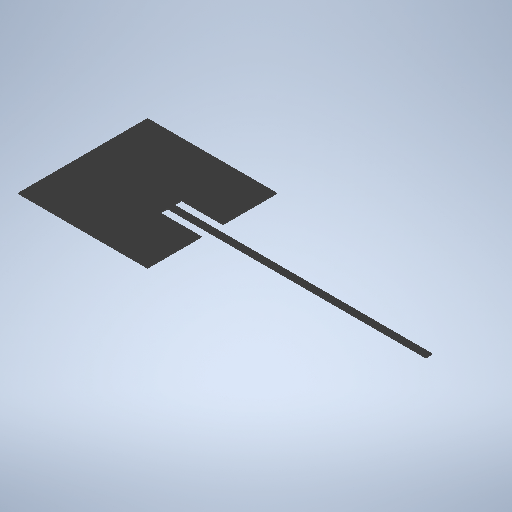
# Autodesk Inventor part: Part17
Saved by Autodesk Inventor 2025.2 (Build 292293000, 293)
## iProperties
Created: 2026-03-30
Part Number: Part17
Material: Generic
Document SubType Name: Modeling
Designer: composite
Density: 1 g/cm^3
Appearance: Default
Author: composite
Autodesk Inventor part; units mm, degrees
ref_plane "YZ Plane" through (0, 0, 0) normal (1, 0, 0) x (0, 1, 0)
ref_plane "XZ Plane" through (0, 0, 0) normal (0, 1, 0) x (-1, 0, 0)
ref_plane "XY Plane" through (0, 0, 0) normal (0, 0, 1) x (1, 0, 0)
sketch "Sketch1" plane through (0, 0, 0) normal (0, 1, 0) x (-1, 0, 0)
  line L0 (0, 0) -> (0, 0.6)
  line L1 (0, 0.6) -> (50, 0.6)
  line L2 (50, 0.6) -> (50, 2.1)
  line L3 (50, 2.1) -> (42, 2.1)
  line L4 (42, 2.1) -> (42, 12.5)
  line L5 (42, 12.5) -> (67, 12.5)
  line L6 (67, 12.5) -> (67, 0)
  line L7 (67, 0) -> (0, 0)
  line L8 (0, 0) -> (0, -0.6)
  line L9 (0, -0.6) -> (50, -0.6)
  line L10 (50, -0.6) -> (50, -2.1)
  line L11 (50, -2.1) -> (42, -2.1)
  line L12 (42, -2.1) -> (42, -12.5)
  line L13 (42, -12.5) -> (67, -12.5)
  line L14 (67, -12.5) -> (67, 0)
  dimension "d1" = 0.6
  dimension "d2" = 50
  dimension "d3" = 1.5
  dimension "d4" = 12.5
  dimension "d5" = 25
  dimension "d6" = 8
  constraints: 30 end point, 6 symmetric about line, 4 perpendicular, 2 vertical, 1 horizontal, 1 horizontal alignment, 1 parallel
  measures "d1" distance of L0.start L0.end
  measures "d2" distance of L0.end L1.end
  measures "d3" distance of L1.end L2.end
  measures "d4" distance of L5.end L6.end
  measures "d5" distance of L4.end L5.end
  measures "d6" distance of L2.end L3.end
extrude "Extrusion1" add sketch "Sketch1" along normal blind 0.1
body "Solid1"
